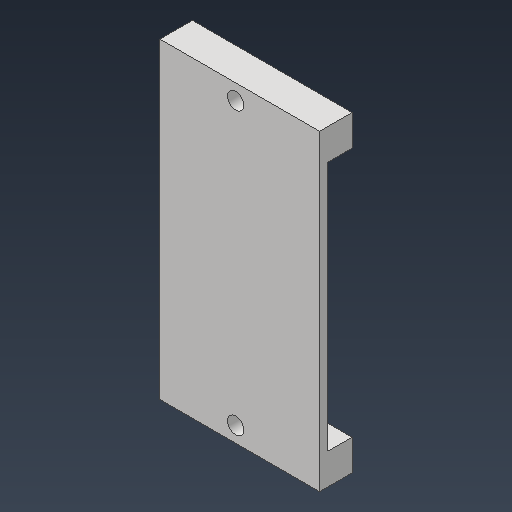
# Autodesk Inventor part: PCBDownlHold
Saved by Autodesk Inventor 2027.1 (Build 311270010, 270A)
## iProperties
Created: 2026-09-08
Part Number: PCBDownlHold
Material: Generic
Document SubType Name: Modeling
Designer: szymo
Density: 1 g/cm^3
Appearance: Default
Author: szymo
Autodesk Inventor part; units mm, degrees
ref_plane "YZ Plane" through (0, 0, 0) normal (1, 0, 0) x (0, 1, 0)
ref_plane "XZ Plane" through (0, 0, 0) normal (0, 1, 0) x (-1, 0, 0)
ref_plane "XY Plane" through (0, 0, 0) normal (0, 0, 1) x (1, 0, 0)
sketch "Sketch1" plane through (0, 0, 0) normal (0, 0, 1) x (1, 0, 0)
  line L0 (1, -38.4) -> (1, -34.6) projected
  line L1 (1, -38.4) -> (20.6442, -38.4) projected
  line L2 (20.6442, -38.4) -> (20.6442, -34.6) projected
  line L3 (1, -34.6) -> (20.6442, -34.6) projected
  circle A0 centre (10.3221, -36.5) radius 1.0065 projected
  line L4 (1, 0) -> (1, -3.8) projected
  line L5 (1, -3.8) -> (20.6442, -3.8) projected
  line L6 (20.6442, 0) -> (20.6442, -3.8) projected
  line L7 (1, 0) -> (20.6442, 0) projected
  circle A1 centre (10.3221, -1.9) radius 1.0065 projected
  point P0 (0, 0)
extrude "Extrusion1" add sketch "Sketch1" along normal blind 4
sketch "Sketch2" plane through (0, 0, 4) normal (0, 0, 1) x (1, 0, 0)
  line L0 (20.6442, -34.6) -> (1, -34.6) projected
  line L1 (1, -34.6) -> (1, -38.4) projected
  line L2 (1, -38.4) -> (20.6442, -38.4) projected
  line L3 (20.6442, -38.4) -> (20.6442, -34.6) projected
  circle A0 centre (10.3221, -36.5) radius 1.0065 projected
  line L4 (1, 0) -> (1, -3.8) projected
  line L5 (1, -3.8) -> (20.6442, -3.8) projected
  line L6 (20.6442, -3.8) -> (20.6442, 0) projected
  line L7 (20.6442, 0) -> (1, 0) projected
  circle A1 centre (10.3221, -1.9) radius 1.0065 projected
  line L8 (1, -34.6) -> (1, -3.8)
  line L9 (20.6442, -3.8) -> (20.6442, -34.6)
  point P0 (0, 0)
  constraints: 4 end point, 1 collinear, 1 parallel
extrude "Extrusion2" add sketch "Sketch2" against normal blind 1 contours L0 L8 L5 L9
body "Solid1"
